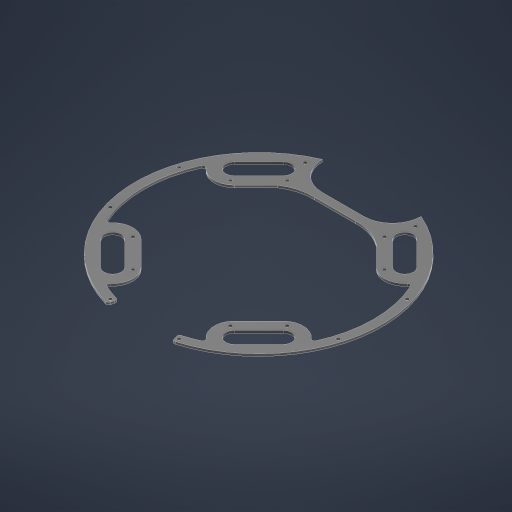
# Autodesk Inventor part: MettalringUnten_v3
Saved by Autodesk Inventor 2023 (Build 270158000, 158)
## iProperties
Created: 2022-10-10
Part Number: MettalringUnten_v3
Material: Generic
Document SubType Name: Modeling
Designer: braun
Density: 1 g/cm^3
Appearance: Smooth - Black
Author: braun
Autodesk Inventor part; units mm, degrees
ref_plane "YZ Plane" through (0, 0, 0) normal (1, 0, 0) x (0, 1, 0)
ref_plane "XZ Plane" through (0, 0, 0) normal (0, 1, 0) x (-1, 0, 0)
ref_plane "XY Plane" through (0, 0, 0) normal (0, 0, 1) x (1, 0, 0)
sketch "Sketch1" plane through (0, 0, 0) normal (0, 1, 0) x (-1, 0, 0)
  circle A0 centre (0, 0) radius 110 construction
  arc A1 (43.0581, -98.5) -> (-43.0581, -98.5) centre (0, 0) ccw
  line L0 (0, -107.5) -> (0, -98.5) construction
  line L1 (0, -98.5) -> (0, -73.5) construction
  line L2 (0, -98.5) -> (-43.0581, -98.5) construction
  line L3 (0, -98.5) -> (43.0581, -98.5) construction
  line L4 (43.0581, -98.5) -> (-43.0581, -98.5) construction
  line L5 (-18.0581, -73.5) -> (18.0581, -73.5)
  arc A2 (43.0581, -98.5) -> (18.0581, -73.5) centre (18.0581, -98.5) ccw
  arc A3 (-18.0581, -73.5) -> (-43.0581, -98.5) centre (-18.0581, -98.5) ccw
  line L6 (0, 107.5) -> (0, 97.5) construction
  line L7 (0, 97.5) -> (-22.5, 97.5) construction
  line L8 (-22.5, 97.5) -> (-22.5, 82.5) construction
  line L9 (22.5, 82.5) -> (22.5, 97.5) construction
  line L10 (22.5, 90) -> (-22.5, 90) construction
  line L11 (15, 97.5) -> (-15, 97.5)
  line L12 (-15, 82.5) -> (15, 82.5)
  arc A4 (15, 82.5) -> (15, 97.5) centre (15, 90) ccw
  arc A5 (-15, 97.5) -> (-15, 82.5) centre (-15, 90) ccw
  line L13 (22.5, 82.5) -> (17.5, 82.5) construction
  line L14 (17.5, 82.5) -> (17.5, 77.5) construction
  circle A6 centre (17.5, 77.5) radius 1.6
  circle A7 centre (-17.5, 77.5) radius 1.6
  line L15 (-58.3363, 79.5495) -> (-79.5495, 58.3363)
  arc A8 (-47.7297, 68.9429) -> (-58.3363, 79.5495) centre (-53.033, 74.2462) ccw
  arc A9 (-79.5495, 58.3363) -> (-68.9429, 47.7297) centre (-74.2462, 53.033) ccw
  line L16 (-68.9429, 47.7297) -> (-47.7297, 68.9429)
  circle A10 centre (-67.1751, 42.4264) radius 1.6
  circle A11 centre (-42.4264, 67.1751) radius 1.6
  line L17 (-97.5, 15) -> (-97.5, -15)
  arc A12 (-82.5, 15) -> (-97.5, 15) centre (-90, 15) ccw
  arc A13 (-97.5, -15) -> (-82.5, -15) centre (-90, -15) ccw
  line L18 (-82.5, -15) -> (-82.5, 15)
  circle A14 centre (-77.5, -17.5) radius 1.6
  circle A15 centre (-77.5, 17.5) radius 1.6
  line L19 (-79.5495, -58.3363) -> (-58.3363, -79.5495)
  arc A16 (-68.9429, -47.7297) -> (-79.5495, -58.3363) centre (-74.2462, -53.033) ccw
  arc A17 (-58.3363, -79.5495) -> (-47.7297, -68.9429) centre (-53.033, -74.2462) ccw
  line L20 (-47.7297, -68.9429) -> (-68.9429, -47.7297)
  circle A18 centre (-42.4264, -67.1751) radius 1.6
  circle A19 centre (-67.1751, -42.4264) radius 1.6
  line L21 (-15, -97.5) -> (15, -97.5)
  arc A20 (-15, -82.5) -> (-15, -97.5) centre (-15, -90) ccw
  arc A21 (15, -97.5) -> (15, -82.5) centre (15, -90) ccw
  line L22 (15, -82.5) -> (-15, -82.5)
  circle A22 centre (17.5, -77.5) radius 1.6
  circle A23 centre (-17.5, -77.5) radius 1.6
  line L23 (58.3363, -79.5495) -> (79.5495, -58.3363)
  arc A24 (47.7297, -68.9429) -> (58.3363, -79.5495) centre (53.033, -74.2462) ccw
  arc A25 (79.5495, -58.3363) -> (68.9429, -47.7297) centre (74.2462, -53.033) ccw
  line L24 (68.9429, -47.7297) -> (47.7297, -68.9429)
  circle A26 centre (67.1751, -42.4264) radius 1.6
  circle A27 centre (42.4264, -67.1751) radius 1.6
  line L25 (97.5, -15) -> (97.5, 15)
  arc A28 (82.5, -15) -> (97.5, -15) centre (90, -15) ccw
  arc A29 (97.5, 15) -> (82.5, 15) centre (90, 15) ccw
  line L26 (82.5, 15) -> (82.5, -15)
  circle A30 centre (77.5, 17.5) radius 1.6
  circle A31 centre (77.5, -17.5) radius 1.6
  line L27 (79.5495, 58.3363) -> (58.3363, 79.5495)
  arc A32 (68.9429, 47.7297) -> (79.5495, 58.3363) centre (74.2462, 53.033) ccw
  arc A33 (58.3363, 79.5495) -> (47.7297, 68.9429) centre (53.033, 74.2462) ccw
  line L28 (47.7297, 68.9429) -> (68.9429, 47.7297)
  circle A34 centre (42.4264, 67.1751) radius 1.6
  circle A35 centre (67.1751, 42.4264) radius 1.6
  line L29 (58.3363, -58.3363) -> (51.2652, -51.2652) construction
  line L30 (40.6586, -61.8718) -> (61.8718, -40.6586)
  arc A36 (40.6586, -61.8718) -> (44.5267, -89.5398) centre (53.033, -74.2462) ccw
  arc A37 (89.5398, -44.5267) -> (61.8718, -40.6586) centre (74.2462, -53.033) ccw
  line L31 (0, -73.5) -> (0, -66.5) construction
  arc A38 (44.5267, 89.5398) -> (40.6586, 61.8718) centre (53.033, 74.2462) ccw
  line L32 (61.8718, 40.6586) -> (40.6586, 61.8718)
  arc A39 (61.8718, 40.6586) -> (89.5398, 44.5267) centre (74.2462, 53.033) ccw
  arc A40 (-89.5398, 44.5267) -> (-61.8718, 40.6586) centre (-74.2462, 53.033) ccw
  line L33 (-40.6586, 61.8718) -> (-61.8718, 40.6586)
  arc A41 (-40.6586, 61.8718) -> (-44.5267, 89.5398) centre (-53.033, 74.2462) ccw
  arc A42 (-44.5267, -89.5398) -> (-40.6586, -61.8718) centre (-53.033, -74.2462) ccw
  line L34 (-61.8718, -40.6586) -> (-40.6586, -61.8718)
  arc A43 (-61.8718, -40.6586) -> (-89.5398, -44.5267) centre (-74.2462, -53.033) ccw
  arc A44 (89.5398, -44.5267) -> (89.5398, 44.5267) centre (0, 0) ccw
  arc A45 (44.5267, 89.5398) -> (-44.5267, 89.5398) centre (0, 0) ccw
  arc A46 (-89.5398, 44.5267) -> (-89.5398, -44.5267) centre (0, 0) ccw
  line L35 (43.0581, -98.5) -> (48.0581, -98.5) construction
  line L36 (48.0581, -98.5) -> (48.0581, -88.5) construction
  circle A47 centre (48.0581, -88.5) radius 1.6
  circle A48 centre (-48.0581, -88.5) radius 1.6
  line L37 (18.0581, -66.5) -> (-18.0581, -66.5)
  arc A49 (17.5, -66.5) -> (43.0581, -59.4724) centre (19.5145, -23.8377) ccw
  arc A50 (-44.5267, -58.0038) -> (-18.0581, -66.5) centre (-19.5089, -25.5422) ccw
  point P0 (0, 90)
  point P1 (-45.9619, 70.7107)
  point P2 (-82.5, 17.5)
  point P3 (-70.7107, -45.9619)
  point P4 (-17.5, -82.5)
  point P5 (45.9619, -70.7107)
  point P6 (82.5, -17.5)
  point P7 (70.7107, 45.9619)
  point P8 (35.7159, -76.7698)
  dimension "d0" = 220
  dimension "d1" = 215
  dimension "d2" = 9
  dimension "d3" = 25
  dimension "d4" = 10
  dimension "d5" = 22.5
  dimension "d6" = 15
  dimension "d7" = 45
  dimension "d8" = 5
  dimension "d9" = 5
  dimension "d10" = 3.2
  dimension "d15" = 86.1162
  dimension "d16" = 45
  dimension "d19" = 360
  dimension "d22" = 10
  dimension "d23" = 7
  dimension "d26" = 360
  dimension "d33" = 5
  dimension "d34" = 10
  dimension "d35" = 3.2
  constraints: 80 end point, 70 point on circle, 51 centre point, 18 point on line, 6 tangent, 5 coincident, 5 midpoint, 4 vertical, 2 horizontal, 2 symmetric about line, 1 collinear, 1 parallel, 1 perpendicular, 160 other
  measures "d0" diameter of A0
  measures "d1" diameter of A1
  measures "d2" distance of L0.start L0.end
  measures "d3" distance of L0.end L1.end
  measures "d4" distance of L6.start L6.end
  measures "d5" distance of L6.end L7.end
  measures "d6" distance of L7.end L8.end
  measures "d7" distance of L8.end L9.start
  measures "d8" distance of L9.start L13.end
  measures "d9" distance of L13.end L14.end
  measures "d10" diameter of A6
  measures "d15" distance of L3.end L2.end
  measures "d16" distance of L10.start L10.end
  measures "d22" distance of L29.start L29.end
  measures "d23" distance of L1.end L31.end
  measures "d33" distance of L3.end L35.end
  measures "d34" distance of L35.end L36.end
  measures "d35" diameter of A47
extrude "Extrusion1" add sketch "Sketch1" along normal blind 2 contours A2 L5 A3 A1
fillet "Fillet2" radius 2 6 edges at (-44.5267, 1, 89.5398) (44.5267, 1, 89.5398) (89.5398, 1, 44.5267) (89.5398, 1, -44.5267) (-89.5398, 1, -44.5267) (-89.5398, 1, 44.5267)
sketch "Sketch4" plane through (0, 2, 0) normal (0, 1, 0) x (1, 0, 0)
  circle A0 centre (0, 0) radius 103.75 construction
  line L0 (0, -103.75) -> (-30, -103.75) construction
  line L1 (-30, -103.75) -> (-30, -99.318) construction
  line L2 (0, -103.75) -> (0, -91.6543) construction
  line L3 (0, 0) -> (-10.2863, 0) construction
  circle A1 centre (-30, -99.318) radius 1.6
  circle A2 centre (30, -99.318) radius 1.6
  circle A3 centre (99.318, -30) radius 1.6
  circle A4 centre (99.318, 30) radius 1.6
  circle A5 centre (-99.318, -30) radius 1.6
  circle A6 centre (-99.318, 30) radius 1.6
  dimension "d45" = 207.5
  dimension "d46" = 30
  dimension "d47" = 3.2
  dimension "d50" = 90
  constraints: 8 end point, 7 centre point, 3 symmetric about line, 2 coincident, 2 horizontal, 2 point on circle, 1 perpendicular, 1 vertical, 8 other
  measures "d45" diameter of A0
  measures "d46" distance of L0.start L0.end
  measures "d47" diameter of A1
extrude "Extrusion4" cut sketch "Sketch4" against normal blind 2
sketch "Sketch5" plane through (0, 2, 0) normal (0, 1, 0) x (1, 0, 0)
  circle A0 centre (0, 0) radius 100
  arc A1 (-41.3697, -91.0415) -> (41.3697, -91.0415) centre (0, 0) ccw projected
  circle A2 centre (0, 0) radius 107.5
  circle A3 centre (-30, -99.318) radius 1.6 construction
  circle A4 centre (-30, -99.318) radius 1.6 construction
  circle A5 centre (30, -99.318) radius 1.6 construction
  circle A6 centre (30, -99.318) radius 1.6 construction
  circle A7 centre (-22.8014, -101.2134) radius 1.6
  arc A8 (-30, -99.318) -> (-22.8014, -101.2134) centre (0, 0) ccw construction
  line L0 (-26.4177, -100.3303) -> (-25.4629, -96.7039) construction
  line L1 (-26.4177, -100.3303) -> (-24.1782, -100.92) construction
  line L2 (-26.4177, -100.3303) -> (-27.3726, -103.9567) construction
  line L3 (0, -100) -> (0, -107.5) construction
  arc A9 (-43.0581, 98.5) -> (43.0581, 98.5) centre (0, 0) ccw construction
  line L4 (-28.3384, -103.6976) -> (-26.4299, -96.4493)
  line L5 (-26.4299, -96.4493) -> (-24.4958, -96.9585) construction
  line L6 (-24.4958, -96.9585) -> (-26.4044, -104.2068)
  line L7 (-26.4055, -104.2113) -> (-28.3396, -103.7021) construction
  line L8 (-28.3396, -103.7021) -> (-24.4958, -96.9585) construction
  line L9 (-26.4299, -96.4493) -> (-26.4055, -104.2113) construction
  line L10 (-26.4299, -96.4493) -> (-26.4286, -96.4444)
  line L11 (-24.4958, -96.9585) -> (-24.4946, -96.9537)
  line L12 (28.3384, -103.6976) -> (26.4299, -96.4493)
  line L13 (24.4958, -96.9585) -> (26.4044, -104.2068)
  line L14 (26.4299, -96.4493) -> (26.4286, -96.4444)
  line L15 (24.4958, -96.9585) -> (24.4946, -96.9537)
  circle A10 centre (22.8014, -101.2134) radius 1.6
  dimension "d54" = 3.2
  dimension "d56" = 90
  dimension "d57" = 90
  dimension "d58" = 2
  constraints: 32 end point, 11 point on circle, 7 centre point, 7 symmetric about line, 5 coincident, 2 midpoint, 2 parallel, 1 concentric, 1 perpendicular, 1 tangent, 1 vertical, 1 other
  measures "d54" diameter of A7
  measures "d56" angle of L0 L1
  measures "d57" angle of L1 L2
  measures "d58" distance of L4.end L5.end
extrude "Extrusion5" cut sketch "Sketch5" against normal blind 10 contours A0 L11 L6 A2 L4 L10 | L14 L12 A2 L13 L15 A0 | A0 L15 L13 A2 L6 L11 | A7 | A10
fillet "Fillet3" radius 2 4 edges at (-28.3384, 1, 103.6976) (-26.4286, 1, 96.4444) (28.3384, 1, 103.6976) (26.4286, 1, 96.4444)
body "Solid1"
